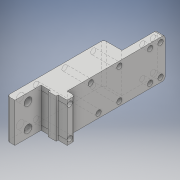
# Autodesk Inventor part: Esteira - estrutura
Saved by Autodesk Inventor 2017 (Build 210142000, 142)
## iProperties
Created: 2020-09-26
Part Number: Esteira - estrutura
Material: Generic
Document SubType Name: Modeling
Designer: ale
Density: 1 g/cm^3
Appearance: Default
Author: ale
Autodesk Inventor part; units mm, degrees
ref_plane "YZ Plane" through (0, 0, 0) normal (1, 0, 0) x (0, 1, 0)
ref_plane "XZ Plane" through (0, 0, 0) normal (0, 1, 0) x (-1, 0, 0)
ref_plane "XY Plane" through (0, 0, 0) normal (0, 0, 1) x (1, 0, 0)
sketch "Sketch1" plane through (0, 0, 0) normal (0, 0, 1) x (1, 0, 0)
  line L0 (0, 0) -> (20, 0)
  line L1 (0, 0) -> (0, -20)
  line L2 (14, 6) -> (20, 6)
  line L3 (0, -20) -> (-6, -20)
  line L4 (20, 6) -> (20, 0)
  line L5 (-6, -20) -> (-6, 54)
  line L6 (14, 6) -> (14, 81)
  line L7 (8, 54) -> (8, 81)
  line L8 (8, 81) -> (14, 81)
  line L9 (8, 54) -> (-6, 54)
  dimension "d1" = 20
  dimension "d3" = 20
  dimension "d7" = 20
  dimension "d8" = 14
  dimension "d9" = 27
  dimension "d46" = 54
  constraints: 20 end point, 3 vertical, 2 horizontal, 1 parallel, 1 perpendicular
  measures "d1" distance of L0.start L1.end
  measures "d3" distance of L0.end L0.start
  measures "d7" distance between parallel lines of L5 L6
  measures "d8" distance of L5.end L7.start
  measures "d9" distance of L7.start L7.end
  measures "d46" distance between parallel lines of L0 L9
extrude "Extrusion1" add sketch "Sketch1" along normal blind 30
sketch "Sketch2" plane through (14, 6, 0) normal (1, 0, 0) x (0, 0, -1)
  line L0 (0, 75) -> (-30, 75) projected
  line L1 (-15, 75) -> (-15, 48)
  line L2 (0, 48) -> (-30, 48) projected
  line L3 (-30, 0) -> (-30, 75) projected
  line L4 (0, 0) -> (0, 75) projected
  line L5 (-30, 67.5) -> (0, 67.5)
  point P0 (0, -6)
  point P1 (-26.5, 71.5)
  point P2 (-3.5, 71.5)
  point P3 (-26.5, 63.5)
  point P4 (-3.5, 63.5)
  dimension "d12" = 3.5
  dimension "d13" = 3.5
  constraints: 4 end point, 3 symmetric about line, 2 midpoint, 2 point on line, 1 perpendicular
  measures "d12" distance from line of point (-26.5, 71.5) L0
  measures "d13" distance from line of point (-26.5, 71.5) L3
hole "Hole1" at (14, 77.5, 26.5) at (14, 77.5, 3.5) at (14, 69.5, 26.5) at (14, 69.5, 3.5) direction (-1, 0, 0) diameter 4 end through all
sketch "Sketch3" plane through (0, 0, 0) normal (0, -1, 0) x (1, 0, 0)
  line L0 (0, 30) -> (20, 30) projected
  line L1 (0, 0) -> (20, 0) projected
  line L2 (13, 30) -> (13, 0)
  line L3 (7, 30) -> (7, 0)
  line L4 (13, 0) -> (7, 0)
  line L5 (7, 30) -> (13, 30)
  constraints: 8 end point, 2 perpendicular
extrude "Extrusion2" add sketch "Sketch3" along normal blind 1.5
sketch "Sketch5" plane through (-6, -20, 0) normal (-1, 0, 0) x (0, 0, 1)
  line L0 (0, 74) -> (30, 74) projected
  line L1 (15, 74) -> (15, 0)
  line L2 (0, 0) -> (30, 0) projected
  line L3 (0, 74) -> (0, 0) projected
  line L4 (15, 44) -> (30, 44)
  line L5 (30, 26) -> (30, 101) projected
  point P0 (0, 20)
  point P1 (3.5, 66)
  point P2 (26.5, 66)
  point P3 (3.5, 22)
  point P4 (26.5, 22)
  point P5 (3.5, 50)
  point P6 (26.5, 44)
  dimension "d26" = 8
  dimension "d27" = 3.5
  dimension "d28" = 30
  constraints: 4 end point, 3 point on line, 3 symmetric about line, 2 midpoint
  measures "d26" distance from line of point (3.5, 66) L0
  measures "d27" distance from line of L3 point (3.5, 66)
  measures "d28" distance of L1.start L4.start
hole "Hole2" at (-6, 46, 3.5) at (-6, 46, 26.5) at (-6, 2, 3.5) at (-6, 2, 26.5) at (-6, 30, 3.5) at (-6, 24, 26.5) direction (1, 0, 0) diameter 4 end through all
sketch "Sketch6" plane through (-6, -20, 0) normal (-1, 0, 0) x (0, 0, 1)
  line L0 (0, 0) -> (30, 0) projected
  line L1 (0, 74) -> (0, 0) projected
  line L2 (15, 0) -> (15, 31.0805)
  point P0 (0, 20)
  point P1 (6, 10)
  point P2 (24, 10)
  dimension "d36" = 10
  dimension "d37" = 6
  constraints: 2 end point, 1 midpoint, 1 symmetric about line, 1 vertical
  measures "d36" distance from line of L0 point (6, 10)
  measures "d37" distance from line of L1 point (6, 10)
hole "Hole3" at (-6, -10, 6) at (-6, -10, 24) direction (1, 0, 0) diameter 6 end through all
fillet "Fillet2" radius 2 5 edges at (-6, -20, 15) (20, 6, 15) (-6, 54, 15) (11, 81, 30) (11, 81, 0)
body "Solid1"
